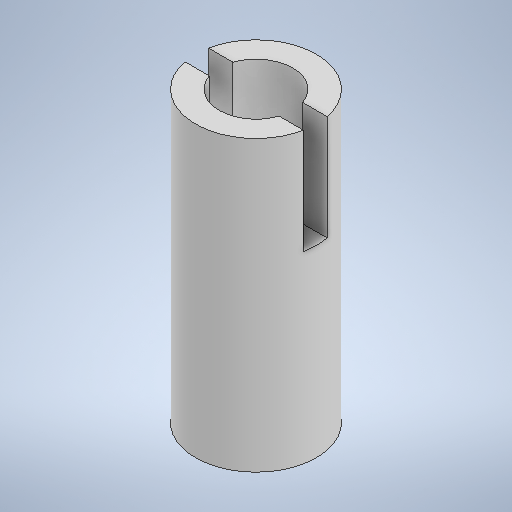
# Autodesk Inventor part: Honigfschleuder Motorkupplung
Saved by Autodesk Inventor 2025 (Build 290162010, 162A)
## iProperties
Created: 2025-11-15
Part Number: Honigfschleuder Motorkupplung
Material: Generisch
Document SubType Name: Modeling
Designer: max-h
Density: 1 g/cm^3
Appearance: Vorgabe
Author: max-h
Autodesk Inventor part; units mm, degrees
ref_plane "YZ Plane" through (0, 0, 0) normal (1, 0, 0) x (0, 1, 0)
ref_plane "XZ Plane" through (0, 0, 0) normal (0, 1, 0) x (-1, 0, 0)
ref_plane "XY Plane" through (0, 0, 0) normal (0, 0, 1) x (1, 0, 0)
sketch "Skizze1" plane through (0, 0, 0) normal (0, 1, 0) x (-1, 0, 0)
  circle A0 centre (0, 0) radius 11.5
  dimension "d0" = 23
  constraints: 1 centre point, 1 coincident
  measures "d0" diameter of A0
extrude "Extrusion1" add sketch "Skizze1" along normal blind 55
sketch "Skizze2" plane through (0, 55, 0) normal (0, 1, 0) x (1, 0, 0)
  circle A0 centre (0, 0) radius 7
  dimension "d3" = 14
  constraints: 1 centre point, 1 coincident
  measures "d3" diameter of A0
extrude "Extrusion2" cut sketch "Skizze2" against normal blind 25
sketch "Skizze3" plane through (0, 55, 0) normal (0, 1, 0) x (1, 0, 0)
  line L0 (12.5, -2.25) -> (-12.5, -2.25)
  line L1 (-12.5, -2.25) -> (-12.5, 2.25)
  line L2 (-12.5, 2.25) -> (12.5, 2.25)
  line L3 (12.5, 2.25) -> (12.5, -2.25)
  line L4 (-17.5, 0) -> (17.5, 0) projected
  line L5 (0, 16.1) -> (0, -16.1) projected
  point P0 (0, 0)
  dimension "d6" = 4.5
  dimension "d7" = 25
  constraints: 8 end point, 2 parallel, 1 horizontal, 1 perpendicular, 2 other
  measures "d6" distance between parallel lines of L2 L0
  measures "d7" distance of L0.start L0.end
extrude "Extrusion3" cut sketch "Skizze3" against normal blind 20
sketch "Skizze4" plane through (0, 0, 0) normal (0, -1, 0) x (1, 0, 0)
  circle A0 centre (0, 0) radius 7.5
  line L0 (-7.0711, -2.5) -> (-9.5, -2.5)
  line L1 (-9.5, -2.5) -> (-9.5, 2.5)
  line L2 (-9.5, 2.5) -> (-7.0711, 2.5)
  line L3 (-7.0711, 2.5) -> (-7.0711, -2.5)
  line L4 (-16.1, 0) -> (16.1, 0) projected
  point P0 (7.5, 0)
  point P1 (-7.0711, 2.5)
  dimension "d10" = 15
  dimension "d12" = 17
  dimension "d13" = 5
  constraints: 8 end point, 2 parallel, 2 point on circle, 1 centre point, 1 coincident, 1 horizontal, 1 perpendicular, 1 point on line, 1 other
  measures "d10" diameter of A0
  measures "d12" distance from line of L1 A0.start
  measures "d13" distance between parallel lines of L2 L0
extrude "Extrusion4" cut sketch "Skizze4" against normal blind 25
